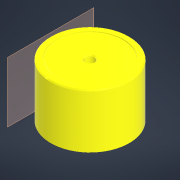
# Autodesk Inventor part: 010
Saved by Autodesk Inventor 2022 (Build 260153000, 153)
## iProperties
Created: 2021-10-31
Part Number: 010
Material: Stainless Steel, 440C
Document SubType Name: Modeling
Designer: vinicius.miguel
Density: 7.75 g/cm^3
Appearance: Smooth - Yellow
Author: vinicius.miguel
Autodesk Inventor part; units mm, degrees
ref_plane "XZ Plane" through (0, 0, 0) normal (0, 1, 0) x (-1, 0, 0)
ref_plane "XY Plane" through (0, 0, 0) normal (0, 0, 1) x (1, 0, 0)
sketch "Sketch1" plane through (0, 0, 0) normal (0, 0, 1) x (1, 0, 0)
  line L0 (-4, 0) -> (-4, 7)
  line L1 (-4, 7) -> (-4.5, 7.5)
  line L2 (-4.5, 7.5) -> (-4.5, 48.5)
  line L3 (-4.5, 48.5) -> (-33, 48.5)
  line L4 (-33, 48.5) -> (-33, 49)
  line L5 (-33, 49) -> (-39, 49)
  line L6 (-33.5, 44) -> (-11, 44)
  line L7 (-11, 44) -> (-11, 3)
  line L8 (-11, 3) -> (-8, 0)
  line L9 (-8, 0) -> (-4, 0)
  line L10 (0, 0) -> (0, 13.1371)
  line L11 (-39, 49) -> (-39, -4.5)
  line L12 (-39, -4.5) -> (-34.5, -4.5)
  line L13 (-34.5, -4.5) -> (-34.5, -5.5)
  line L14 (-34.5, -5.5) -> (-33.5, -5.5)
  line L15 (-33.5, -5.5) -> (-33.5, 44)
  line L16 (-33, 48.5) -> (-33, 48.25)
  line L17 (-33, 48.25) -> (-31.5, 48.5)
  line L18 (-35, -4.5) -> (-34.5, -4.35)
  line L19 (-34.5, -4.35) -> (-34.5, -4.5)
  dimension "d0" = 8
  dimension "d1" = 7
  dimension "d7" = 135
  dimension "d9" = 135
  dimension "d11" = 4.5
  dimension "d12" = 9
  dimension "d13" = 16
  dimension "d14" = 22
  dimension "d15" = 0.5
  dimension "d19" = 44
  dimension "d20" = 66
  dimension "d27" = 6.5
  dimension "d28" = 49
  dimension "d29" = 5
  dimension "d31" = 67
  dimension "d32" = 4.5
  dimension "d34" = 1
  dimension "d35" = 0.25
  dimension "d36" = 1.5
  dimension "d37" = 78
  dimension "d38" = 5.5
  dimension "d39" = 0.15
  dimension "d40" = 0.5
  dimension "d41" = 4.5
  constraints: 40 end point, 8 perpendicular, 4 vertical, 3 parallel, 2 point on line, 1 horizontal alignment
  measures "d0" diameter of L0 L10
  measures "d1" distance of L0.start L0.end
  measures "d7" angle of L7 L8
  measures "d9" angle of L0 L1
  measures "d11" distance between parallel lines of L6 L3
  measures "d12" diameter of L2 L10
  measures "d13" diameter of L8.end L10
  measures "d14" diameter of L7 L10
  measures "d15" distance between parallel lines of L3 L5
  measures "d19" distance between parallel lines of L6 L9
  measures "d20" diameter of L4 L10
  measures "d27" distance between parallel lines of L2 L7
  measures "d28" distance from line of L5 L10.start
  measures "d29" distance between parallel lines of L5 L6
  measures "d31" diameter of L15 L10
  measures "d32" distance of L11.end L12.end
  measures "d34" distance of L12.end L13.end
  measures "d35" distance of L3.end L16.end
  measures "d36" horizontal distance of L17.end L16.end
  measures "d37" diameter of L11 L10
  measures "d38" distance between parallel lines of L11 L15
  measures "d39" distance of L18.end L12.end
  measures "d40" distance of L12.end L18.start
  measures "d41" distance between parallel lines of L12 L9
revolve "Revolution1" add sketch "Sketch1" angle 360 about axis through (0, 0, 0) along (0, 1, 0) contours L9 L8 L7 L6 L15 L14 L13 L19 L18 L12 L11 L5 L4 L16 L17 L3 L2 L1 L0
chamfer "Chamfer1" distance 1 angle 45 1 edges at (4.5, 48.5, 0)
ref_plane "Work Plane1" through (-39, 22.25, 0) normal (1, 0, 0) x (0, 1, 0)
sketch "Sketch2" plane through (-39, 22.25, 0) normal (1, 0, 0) x (0, 1, 0)
  line L0 (-22.75, 0) -> (-37.8891, 0) construction
  line L1 (-22.75, 3) -> (-37.8891, 3)
  line L2 (-37.8891, -3) -> (-22.75, -3)
  arc A0 (-22.75, -3) -> (-22.75, 3) centre (-22.75, 0) ccw
  arc A1 (-37.8891, 3) -> (-37.8891, -3) centre (-37.8891, 0) ccw
  line L3 (-27.75, -34.5) -> (-27.75, 34.5) projected
  point P0 (-22.25, 0)
  point P1 (-30.3196, 0)
  dimension "d42" = 6
  dimension "d43" = 5
  constraints: 8 end point, 4 point on circle, 4 tangent, 2 centre point, 1 horizontal, 1 horizontal alignment, 1 midpoint, 1 parallel
  measures "d42" diameter of A1
  measures "d43" distance from line of L3 L0.start
extrude "Extrusion1" cut sketch "Sketch2" along normal blind 10
chamfer "Chamfer2" distance 1 angle 45 1 edges at (39, 49, 0)
body "Solid1"
